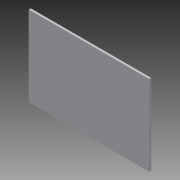
# Autodesk Inventor part: Techo
Saved by Autodesk Inventor 2013 (Build 170138000, 138)
## iProperties
Created: 2015-11-12
Part Number: Techo
Material: Generic
Document SubType Name: Modeling
Designer: serge
Density: 1 g/cm^3
Author: serge
Autodesk Inventor part; units mm, degrees
ref_plane "YZ Plane" through (0, 0, 0) normal (1, 0, 0) x (0, 1, 0)
ref_plane "XZ Plane" through (0, 0, 0) normal (0, 1, 0) x (-1, 0, 0)
ref_plane "XY Plane" through (0, 0, 0) normal (0, 0, 1) x (1, 0, 0)
sketch "Sketch1" plane through (0, 0, 0) normal (0, 1, 0) x (-1, 0, 0)
  line L0 (-5996.8444, -3995.6306) -> (3.1556, -3995.6306)
  line L1 (3.1556, -3995.6306) -> (3.1556, 4.3694)
  line L2 (3.1556, 4.3694) -> (-5996.8444, 4.3694)
  line L3 (-5996.8444, 4.3694) -> (-5996.8444, -3995.6306)
  line L4 (-5996.8444, -3995.6306) -> (3.1556, 4.3694) construction
  line L5 (3.1556, -3995.6306) -> (-5996.8444, 4.3694) construction
  point P0 (0, 0)
  point P1 (-2996.8444, -1995.6306)
  dimension "Largo" = 6000
  dimension "Ancho" = 4000
  constraints: 12 end point, 2 midpoint, 2 parallel, 1 horizontal, 1 perpendicular
  measures "Largo" distance of L1.end L2.end
  measures "Ancho" distance of L0.end L1.end
extrude "Extrusion1" add sketch "Sketch1" along normal blind 101.6
equation "\"Largo\" = T_L"
equation "\"Ancho\" = T_A"
equation "\"Espesor\" = T_E"
equation "\"PE_N\" = 101.6"
equation "\"PE_S\" = 101.6"
equation "\"PE_EO\" = 101.6"
equation "\"T_L\" = 6000"
equation "\"T_A\" = 4000"
equation "\"T_E\" = 101.6"
equation "\"lon_ve\" = 512.5"
equation "\"n_a\" = 3"
equation "\"t_a\" = 19.05"
equation "\"d_a\" = 128.125"
equation "\"lon_ho\" = 749"
equation "\"d_bor\" = 59.92"
equation "\"lon_gui\" = 187.25"
equation "\"esp_gui\" = 461.25"
equation "\"lon_ve2\" = 498.475"
equation "\"n_a2\" = 3"
equation "\"t_a2\" = 124.61875"
equation "\"d_a2\" = 19.05"
equation "\"lon_ho2\" = 933.45"
equation "\"d_bor2\" = 74.676"
equation "\"lon_gui2\" = 233.3625"
equation "\"esp_gui2\" = 448.6275"
body "Solid1"
